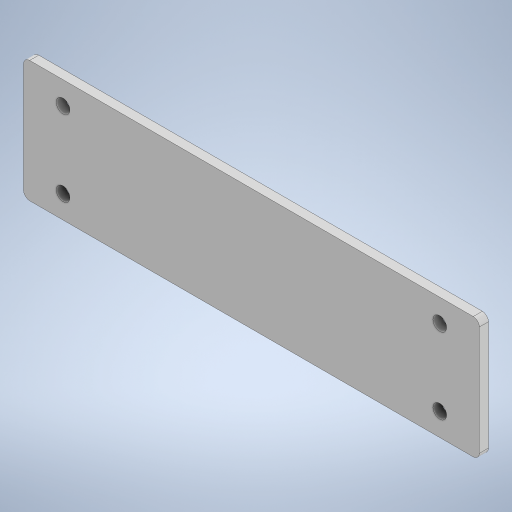
# Autodesk Inventor part: Stabilisator_05
Saved by Autodesk Inventor 2024 (Build 280153000, 153)
## iProperties
Created: 2024-03-25
Part Number: Stabilisator_05
Material: Generisch
Document SubType Name: Modeling
Designer: month
Density: 1 g/cm^3
Appearance: Vorgabe
Author: month
Autodesk Inventor part; units mm, degrees
ref_plane "YZ Plane" through (0, 0, 0) normal (1, 0, 0) x (0, 1, 0)
ref_plane "XZ Plane" through (0, 0, 0) normal (0, 1, 0) x (-1, 0, 0)
ref_plane "XY Plane" through (0, 0, 0) normal (0, 0, 1) x (1, 0, 0)
sketch "Skizze1" plane through (0, 0, 0) normal (0, 1, 0) x (-1, 0, 0)
  line L0 (0, 0) -> (150, 0)
  line L1 (150, 0) -> (150, -40)
  line L2 (150, -40) -> (0, -40)
  line L3 (0, -40) -> (0, 0)
  dimension "d0" = 40
  dimension "d1" = 150
  constraints: 8 end point, 2 parallel, 1 horizontal, 1 perpendicular
  measures "d0" distance of L2.end L0.start
  measures "d1" distance of L1.end L2.end
extrude "Extrusion1" add sketch "Skizze1" along normal blind 3
sketch "Skizze2" plane through (0, 3, 0) normal (0, 1, 0) x (1, 0, 0)
  line L0 (-150, 0) -> (0, 0) projected
  line L1 (-75, 0) -> (-75, 40)
  line L2 (0, 40) -> (-150, 40) projected
  line L3 (-150, 40) -> (-150, 0) projected
  line L4 (-150, 20) -> (0, 20)
  line L5 (0, 0) -> (0, 40) projected
  line L6 (-13, 0) -> (-13, 40) construction
  circle A0 centre (-13, 7.5) radius 2.25
  circle A1 centre (-13, 32.5) radius 2.25
  circle A2 centre (-137, 7.5) radius 2.25
  circle A3 centre (-137, 32.5) radius 2.25
  dimension "d4" = 13
  dimension "d5" = 4.5
  dimension "d6" = 4.5
  dimension "d7" = 25
  constraints: 6 end point, 4 centre point, 4 midpoint, 4 point on line, 3 symmetric about line, 1 perpendicular, 2 other
  measures "d4" distance between parallel lines of L5 L6
  measures "d5" diameter of A1
  measures "d6" diameter of A0
  measures "d7" distance of A0.centre A1.centre
extrude "Extrusion2" cut sketch "Skizze2" against normal blind 3 contours A0 | A1 | A2 | A3
fillet "Rundung1" radius 2 4 edges at (-150, 1.5, 0) (-150, 1.5, -40) (0, 1.5, -40) (0, 1.5, 0)
